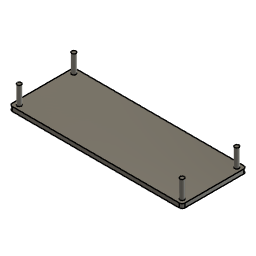
Newkansi v2 (Autodesk Fusion 360 design; units mm, degrees)
Autodesk Fusion 360 part; units mm, degrees
sketch "Sketch1" plane through (0, 0, 0) normal (0, 1, 0) x (1, 0, 0)
  line L0 (0, 0) -> (-123, 0)
  line L1 (-123, 0) -> (-123, 45.95)
  line L2 (-123, 45.95) -> (0, 45.95)
  line L3 (0, 45.95) -> (0, 0)
  dimension "d1" = 123
  dimension "d2" = 45.95
  constraint horizontal L0
  constraint vertical L1
  constraint horizontal L2
  constraint vertical L3
  constraint coincident L0.start L3.end
  measures "d1" distance of L0.start L0.end
  measures "d2" distance of L0.start L2.end
extrude "Extrude1" add sketch "Sketch1" along normal blind 3
sketch "Sketch2" plane through (0, 3, 0) normal (0, 1, 0) x (-1, 0, 0)
  line L0 (0, -45.95) -> (123, -45.95)
  line L1 (123, -45.95) -> (123, 0)
  line L2 (123, 0) -> (0, 0)
  line L3 (0, 0) -> (0, -45.95)
  line L4 (0, 0) -> (5, 0) construction
  line L5 (123, 0) -> (128, 0) construction
  line L6 (123, -45.95) -> (128, -45.95) construction
  line L7 (0, -45.95) -> (5, -45.95) construction
  circle A0 centre (119.4645, -42.4145) radius 1.5
  circle A1 centre (3.5355, -42.4145) radius 1.5
  circle A2 centre (119.4645, -3.5355) radius 1.5
  circle A3 centre (3.5355, -3.5355) radius 1.5
  dimension "d5" = 5
  dimension "d8" = 5
  dimension "d10" = 5
  dimension "d11" = 5
  dimension "d13" = 3
  dimension "d14" = 3
  dimension "d15" = 3
  dimension "d16" = 3
  constraint horizontal L4
  constraint coincident L2.end L3.start
  constraint horizontal L5
  constraint coincident L1.end L2.start
  constraint horizontal L6
  constraint coincident L0.end L1.start
  constraint horizontal L7
  constraint coincident L0.start L3.end
  measures "d5" distance of L2.end A3.centre
  measures "d8" distance of L1.end A2.centre
  measures "d10" distance of L0.end A0.centre
  measures "d11" distance of L0.start A1.centre
  measures "d13" diameter of A0
  measures "d14" diameter of A1
  measures "d15" diameter of A2
  measures "d16" diameter of A3
extrude "Extrude2" add sketch "Sketch2" along normal blind 13 contours A0 | A1 | A2 | A3
fillet "Fillet1" radius 2 2 edges at (-123, 1.5, 0) (0, 1.5, 0)
fillet "Fillet2" radius 2 2 edges at (0, 1.5, -45.95) (-123, 1.5, -45.95)
